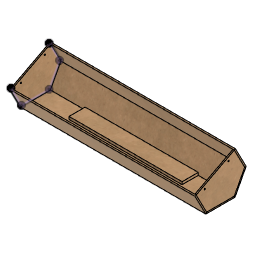
110hp_3u_mdf_case (Autodesk Fusion 360 design; units mm, degrees)
Autodesk Fusion 360 part; units mm, degrees
sketch "Sketch1" plane through (0, 0, 0) normal (1, 0, 0) x (0, 1, 0) in component "Panel1"
  line L0 (-44.8404, -49.3629) -> (40.8096, -49.3629)
  line L1 (40.8096, -49.3629) -> (73.132, 12.0497)
  line L2 (73.132, 12.0497) -> (40.8096, 74.1405)
  line L3 (40.8096, 74.1405) -> (-77.1628, 12.7279)
  line L4 (-77.1628, 12.7279) -> (-44.8404, -49.3629)
  dimension "d7" = 70
  dimension "d8" = 133
  dimension "d9" = 27.5
  constraint horizontal L0
  constraint equal L2 L4
  constraint parallel L2 L4
  constraint perpendicular L2 L3
  constraint vertical L0.end L2.end
  measures "d7" distance of L1.end L2.end
  measures "d8" distance of L2.end L3.end
  measures "d9" angle of L0 L3
extrude "Extrude1" add sketch "Sketch1" along normal blind 4 makes body 1 in component "Panel1"
sketch "Sketch2" plane through (0, 0, 0) normal (-1, 0, 0) x (0, -1, 0) in component "Panel1"
  line L0 (44.8404, -49.3629) -> (77.1628, 12.7279)
  line L1 (77.1628, 12.7279) -> (-40.8096, 74.1405)
  line L2 (-40.8096, 74.1405) -> (-73.132, 12.0497)
  line L3 (-73.132, 12.0497) -> (-40.8096, -49.3629)
  line L4 (-40.8096, -49.3629) -> (44.8404, -49.3629)
  circle A0 centre (-23.2518, 53.7266) radius 2
  circle A1 centre (50.3701, 15.4015) radius 2
  dimension "d12" = 4
  dimension "d13" = 10
  dimension "d14" = 25
  dimension "d15" = 10
  dimension "d16" = 25
  constraint equal A0 A1
  measures "d12" diameter of A0
  measures "d13" distance of L1 A0.centre
  measures "d14" distance of L2 A0.centre
  measures "d15" distance of L1 A1.centre
  measures "d16" distance of L0 A1.centre
extrude "Extrude2" cut sketch "Sketch2" against normal through all contours A0 | A1 bodies 1 in component "Panel1"
sketch "Sketch1 (2)" plane through (0, 0, 0) normal (-1, 0, 0) x (0, -1, 0) in component "Case"
  line L0 (44.8404, -49.3629) -> (77.1628, 12.7279)
  line L1 (-40.8096, 74.1405) -> (-73.132, 12.0497)
  line L2 (-73.132, 12.0497) -> (-40.8096, -49.3629)
  line L3 (-40.8096, -49.3629) -> (44.8404, -49.3629)
  line L4 (-44.3576, 75.9875) -> (-77.6468, 12.0395)
  line L5 (-77.6468, 12.0395) -> (-43.2245, -53.3629)
  line L6 (-43.2245, -53.3629) -> (47.2677, -53.3629)
  line L7 (47.2677, -53.3629) -> (80.7109, 10.8809)
  line L8 (-44.3576, 75.9875) -> (-40.8096, 74.1405)
  line L9 (77.1628, 12.7279) -> (80.7109, 10.8809)
  line L10 (44.8404, -49.3629) -> (47.2677, -53.3629)
  line L11 (-40.8096, -49.3629) -> (-43.2245, -53.3629)
  line L12 (-73.132, 12.0497) -> (-77.6468, 12.0395)
  dimension "d22" = 4
  constraint coincident L1.start L8.end
  constraint perpendicular L1 L8
  constraint coincident L0.end L9.start
  constraint perpendicular L7 L9
  constraint coincident L0.start L3.end
  constraint coincident L2.end L3.start
  constraint coincident L1.end L2.start
extrude "Extrude1'" add sketch "Sketch1 (2)" against normal blind 573 separate body contours L1 L4 L8 L12 makes body 2 in component "Case"
extrude "Extrude2'" add sketch "Sketch1 (2)" against normal blind 573 separate body contours L2 L5 L11 L12 makes body 3 in component "Case"
extrude "Extrude3" add sketch "Sketch1 (2)" against normal blind 573 separate body contours L3 L6 L10 L11 makes body 4 in component "Case"
extrude "Extrude4" add sketch "Sketch1 (2)" against normal blind 573 separate body contours L0 L7 L9 L10 makes body 5 in component "Case"
sketch "Sketch2 (2)" plane through (0, 0, -49.3629) normal (0, 0, 1) x (-1, 0, 0) in component "Case"
  line L0 (0, -40.8096) -> (0, 44.8404)
  line L1 (0, 44.8404) -> (-573, 44.8404)
  line L2 (-573, 44.8404) -> (-573, -40.8096)
  line L3 (-573, -40.8096) -> (0, -40.8096)
  line L4 (-111.5, -40.8096) -> (-461.5, -40.8096)
  line L5 (-461.5, -40.8096) -> (-461.5, 9.1904)
  line L6 (-461.5, 9.1904) -> (-111.5, 9.1904)
  line L7 (-111.5, 9.1904) -> (-111.5, -40.8096)
  line L8 (-4, -40.8096) -> (-4, 77.1628)
  dimension "d31" = 107.5
  dimension "d32" = 350
  dimension "d33" = 50
  constraint horizontal L4
  constraint vertical L5
  constraint horizontal L6
  constraint vertical L7
  constraint collinear L3 L4
  measures "d31" distance of L7 L8
  measures "d32" distance of L5.end L6.end
  measures "d33" distance of L4.end L5.end
extrude "Extrude5" add sketch "Sketch2 (2)" along normal blind 8 separate body contours L3 L4 L5 L6 L7 makes body 6 in component "Case"
component "Panel1" placed x (1, 0, 0) y (0, 1, 0) z (0, 0, 1) at (569, 0, 0)
component "Panel1" placed x (1, 0, 0) y (0, 1, 0) z (0, 0, 1) at (0, 0, 0)
component "Case" placed x (1, 0, 0) y (0, 1, 0) z (0, 0, 1) at (0, 0, 0)
equation "FrameX = 565 mm"
equation "FrameY = 133 mm"
equation "ModuleDepth = 70 mm"
equation "Angle = 27.5 deg"
equation "Thickness = 4 mm"
equation "d7 = ModuleDepth"
equation "d8 = FrameY"
equation "d9 = Angle"
equation "d10 = Thickness"
equation "d21 = Thickness + FrameX"
equation "d22 = Thickness"
equation "d23 = -( Thickness * 2 + FrameX )"
equation "d25 = -( Thickness * 2 + FrameX )"
equation "d27 = -( Thickness * 2 + FrameX )"
equation "d29 = -( Thickness * 2 + FrameX )"
equation "d31 = FrameX / 2 - ( 350 / 2 ) * 1 mm"
